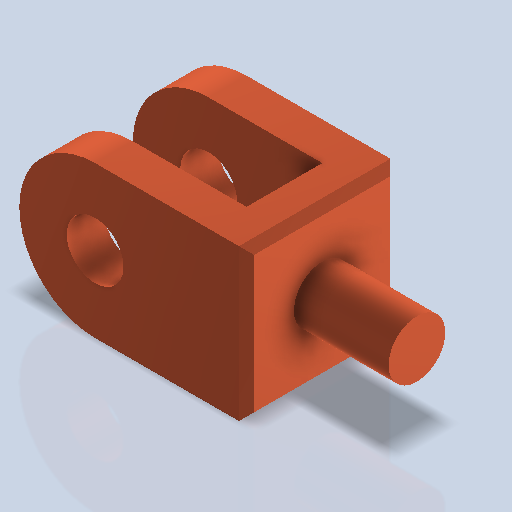
# Autodesk Inventor part: 6
Saved by Autodesk Inventor 2024.2 (Build 282272000, 272)
## iProperties
Created: 2024-05-04
Part Number: 6
Material: Kupfer, Legierung
Document SubType Name: Modeling
Designer: Fabri
Density: 8.92 g/cm^3
Appearance: Kupfer - satiniert
Author: Fabri
Autodesk Inventor part; units mm, degrees
ref_plane "YZ Plane" through (0, 0, 0) normal (1, 0, 0) x (0, 1, 0)
ref_plane "XZ Plane" through (0, 0, 0) normal (0, 1, 0) x (-1, 0, 0)
ref_plane "XY Plane" through (0, 0, 0) normal (0, 0, 1) x (1, 0, 0)
sketch "Skizze1" plane through (0, 0, 0) normal (0, 1, 0) x (-1, 0, 0)
  line L0 (0, 20) -> (40, 20)
  line L1 (40, -20) -> (0, -20)
  line L2 (0, -20) -> (0, 20)
  arc A0 (40, -20) -> (40, 20) centre (40, 0) ccw
  line L3 (0, 0) -> (81.992, 0) construction
  point P0 (20, -20)
  dimension "d0" = 40
  dimension "d2" = 40
  dimension "d3" = 20
  constraints: 8 end point, 2 horizontal, 2 midpoint, 2 point on circle, 2 tangent, 1 centre point, 1 coincident, 1 horizontal alignment, 1 parallel, 1 vertical alignment
  measures "d0" distance from line of point (20, -20) L0
  measures "d2" distance from line of L2 A0.centre
  measures "d3" radius of A0
extrude "Extrusion1" add sketch "Skizze1" along normal blind 40
sketch "Skizze2" plane through (0, 0, 0) normal (0, -1, 0) x (1, 0, 0)
  arc A0 (-40, 20) -> (-40, -20) centre (-40, 0) ccw projected
  point P0 (0, 0)
  constraints: 1 coincident
hole "Bohrung1" at (-40, 0, 0) direction (0, 1, 0) diameter 15 depth 40
sketch "Skizze3" plane through (-40, 0, 20) normal (0, 0, 1) x (1, 0, 0)
  line L0 (30, 10) -> (-20.9704, 10)
  line L1 (-20.9704, 10) -> (-20.9704, 30)
  line L2 (-20.9704, 30) -> (30, 30)
  line L3 (30, 30) -> (30, 10)
  line L4 (40, 0) -> (40, 40) projected
  point P0 (30, 20)
  point P1 (40, 20)
  dimension "d13" = 10
  dimension "d14" = 20
  constraints: 8 end point, 2 midpoint, 2 parallel, 1 horizontal, 1 horizontal alignment, 1 perpendicular
  measures "d13" distance between parallel lines of L4 L3
  measures "d14" distance between parallel lines of L2 L0
extrude "Extrusion2" cut sketch "Skizze3" against normal up to surface (40 mm away)
chamfer "Fasen1" distance 2 angle 45 4 edges at (0, 20, 20) (0, 40, 0) (0, 20, -20) (0, 0, 0)
sketch "Skizze4" plane through (0, 2, -18) normal (1, 0, 0) x (0, 0, -1)
  circle A0 centre (-18, 18) radius 7.5
  line L0 (0, 36) -> (0, 0) projected
  line L1 (-38, -2) -> (2, -2) projected
  point P0 (-18, -2)
  point P1 (0, 18)
  point P2 (-18, -2)
  dimension "d20" = 15
  constraints: 2 midpoint, 1 centre point, 1 horizontal alignment, 1 vertical alignment
  measures "d20" diameter of A0
extrude "Extrusion3" add sketch "Skizze4" along normal blind 25
